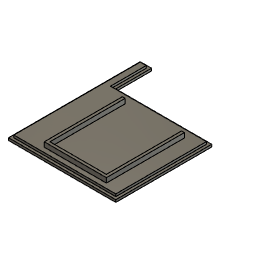
lid v2 (Autodesk Fusion 360 design; units mm, degrees)
Autodesk Fusion 360 part; units mm, degrees
sketch "Sketch1" plane through (0, 0, 0) normal (0, 1, 0) x (1, 0, 0)
  line L0 (67, -50) -> (-47, -50)
  line L1 (-47, -50) -> (-47, 90)
  line L2 (-47, 90) -> (-35, 90)
  line L3 (-35, 90) -> (-35, 52)
  line L4 (-35, 52) -> (67, 52)
  line L5 (67, 52) -> (67, -50)
  line L6 (65.2, -48.2) -> (-45.2, -48.2)
  line L7 (-45.2, -48.2) -> (-45.2, 88.2)
  line L8 (-45.2, 88.2) -> (-36.8, 88.2)
  line L9 (-36.8, 88.2) -> (-36.8, 50.2)
  line L10 (-36.8, 50.2) -> (65.2, 50.2)
  line L11 (65.2, 50.2) -> (65.2, -48.2)
  dimension "d1" = 102
  dimension "d3" = 140
  dimension "d4" = 12
  dimension "d5" = 102
  dimension "d6" = 1.8
  constraint horizontal L0
  constraint perpendicular L0 L1
  constraint perpendicular L1 L2
  constraint perpendicular L2 L3
  constraint perpendicular L3 L4
  constraint perpendicular L0 L5
  measures "d1" distance of L0.start L4.end
  measures "d3" distance of L0.end L1.end
  measures "d4" distance of L1.end L2.end
  measures "d5" distance of L3.end L4.end
extrude "Extrude1" add sketch "Sketch1" along normal blind 2.5 contours L0 L1 L2 L3 L4 L5 | L6 L7 L8 L9 L10 L11
sketch "Sketch2" plane through (0, 2.5, 0) normal (0, 1, 0) x (-1, 0, 0)
  line L0 (-67, -52) -> (35, -52)
  line L1 (35, -52) -> (35, -90)
  line L2 (35, -90) -> (47, -90)
  line L3 (47, -90) -> (47, 50)
  line L4 (47, 50) -> (-67, 50)
  line L5 (-67, 50) -> (-67, -52)
  line L6 (37.8, -87.2) -> (44.2, -87.2)
  line L7 (44.2, -87.2) -> (44.2, 47.2)
  line L8 (44.2, 47.2) -> (-64.2, 47.2)
  line L9 (-64.2, 47.2) -> (-64.2, -49.2)
  line L10 (-64.2, -49.2) -> (37.8, -49.2)
  line L11 (37.8, -49.2) -> (37.8, -87.2)
  dimension "d9" = -2.8
extrude "Extrude2" add sketch "Sketch2" along normal blind 2.5 contours L6 L7 L8 L9 L10 L11
sketch "Sketch3" plane through (0, 5, 0) normal (0, 1, 0) x (-1, 0, 0)
  line L0 (37.8, -49.2) -> (37.8, -87.2)
  line L1 (37.8, -87.2) -> (44.2, -87.2)
  line L2 (44.2, -87.2) -> (44.2, 47.2)
  line L3 (44.2, 47.2) -> (-64.2, 47.2)
  line L4 (-64.2, 47.2) -> (-64.2, -49.2)
  line L5 (-64.2, -49.2) -> (37.8, -49.2)
  line L6 (16.8, -40.8) -> (16.8, 42.2)
  line L7 (16.8, 42.2) -> (-49.2, 42.2)
  line L8 (-49.2, 42.2) -> (-49.2, -40.8)
  line L9 (-49.2, -40.8) -> (-46.2, -40.8)
  line L10 (-46.2, -40.8) -> (-46.2, 39.2)
  line L11 (-46.2, 39.2) -> (13.8, 39.2)
  line L12 (13.8, 39.2) -> (13.8, -40.8)
  line L13 (13.8, -40.8) -> (16.8, -40.8)
  dimension "d12" = 60
  dimension "d13" = 80
  dimension "d14" = 3
  dimension "d15" = 3
  dimension "d16" = 3
  dimension "d17" = 5
  dimension "d18" = 15
  constraint parallel L2 L6
  constraint perpendicular L6 L7
  constraint perpendicular L7 L8
  constraint perpendicular L8 L9
  constraint perpendicular L9 L10
  constraint perpendicular L8 L11
  constraint perpendicular L11 L12
  constraint perpendicular L6 L13
  constraint collinear L9 L13
  measures "d12" distance of L10 L12
  measures "d13" distance of L9 L11
  measures "d14" distance of L6 L12
  measures "d15" distance of L8 L10
  measures "d16" distance of L7 L11
  measures "d17" distance of L3 L7
  measures "d18" distance of L4 L8
extrude "Extrude3" add sketch "Sketch3" along normal blind 5 contours L6 L7 L8 L9 L10 L11 L12 L13
equation "d15 = d14"
equation "d16 = d14"
